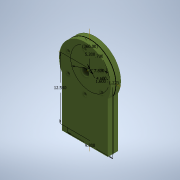
# Autodesk Inventor part: bearing stand
Saved by Autodesk Inventor 2021.1 (Build 251245000, 245)
## iProperties
Created: 2020-08-29
Part Number: bearing stand
Material: Aluminum 6061
Document SubType Name: Sheet Metal
Designer: Vamshi
Mass: 13726.4 g
Surface Area: 2891.24 cm^2
Volume: 5083.86 cm^3
Density: 2.7 g/cm^3
Sheet Metal Rule: Default
Appearance: Dark Olive Green
Author: Vamshi
Autodesk Inventor part; units mm, degrees
ref_plane "YZ Plane" through (0, 0, 0) normal (1, 0, 0) x (0, 1, 0)
ref_plane "XZ Plane" through (0, 0, 0) normal (0, 1, 0) x (-1, 0, 0)
ref_plane "XY Plane" through (0, 0, 0) normal (0, 0, 1) x (1, 0, 0)
sketch "Sketch1" plane through (0, 0, 0) normal (0, 0, 1) x (1, 0, 0)
  circle A0 centre (0, 0) radius 99.06
  line L0 (-116.84, -317.5) -> (116.84, -317.5)
  line L1 (-116.84, -317.5) -> (116.84, -317.5)
  line L2 (-116.84, -317.5) -> (-116.84, -61.5917)
  line L3 (116.84, -317.5) -> (116.84, -61.5917)
  arc A1 (116.84, -61.5917) -> (-116.84, -61.5917) centre (0, 0) ccw
  circle A2 centre (0, 99.06) radius 8.89
  circle A3 centre (-85.7885, 49.53) radius 8.89
  circle A4 centre (-85.7885, -49.53) radius 8.89
  circle A5 centre (0, -99.06) radius 8.89
  circle A6 centre (85.7885, -49.53) radius 8.89
  circle A7 centre (85.7885, 49.53) radius 8.89
  circle A8 centre (0, 0) radius 20.32
  point P0 (0, -317.5)
  dimension "d1" = 198.12
  dimension "d8" = 17.78
  dimension "d11" = 360
  dimension "d13" = 40.64
  dimension "d16" = 132.08
  dimension "d17" = 233.68
  dimension "d18" = 116.84
  dimension "d19" = 317.5
  dimension "d20" = 31.0515
  constraints: 8 centre point, 8 end point, 3 coincident, 2 equal length, 2 point on circle, 1 horizontal, 1 midpoint, 1 vertical, 1 vertical alignment, 15 other
  measures "d8" diameter of A2
  measures "d13" diameter of A8
  measures "d16" radius of A1
  measures "d17" distance between parallel lines of L3 L2
  measures "d18" distance from line of point (0, 0) L3
  measures "d19" distance from line of point (0, 0) L1
  measures "d20" distance from line of A7.centre L3
extrude "Extrusion1" add sketch "Sketch1" along normal mid plane 25.4 contours A0 A6 A5 A4 A3 A2 A7 | L2 A1 L3 L0
sketch "Sketch2" plane through (0, 0, 12.7) normal (0, 0, 1) x (1, 0, 0)
  point P0 (0, 0)
extrude "Extrusion2" add sketch "Sketch1" along normal mid plane 50.8 contours A0 A6 A5 A4 A3 A2 A7 | L2 A1 L3 L0
equation "\"BendRadius\" = Thickness"
equation "\"BendReliefWidth\" = Thickness"
equation "\"BendReliefDepth\" = 0.5 * Thickness"
equation "\"CornerReliefSize\" = 4 * Thickness"
equation "\"MinimumRemnant\" = 2 * Thickness"
equation "\"TransitionRadius\" = BendRadius"
equation "\"JacobiRadiusSize\" = BendRadius"
equation "\"GapSize\" = Thickness"
equation "\"Thickness\" = 3.048"
body "Solid1"
